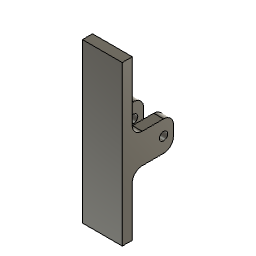
Basis v1 (Autodesk Fusion 360 design; units mm, degrees)
Autodesk Fusion 360 part; units mm, degrees
sketch "Skizze1" plane through (0, 0, 0) normal (1, 0, 0) x (0, 1, 0)
  line L0 (-16.5, 79.8295) -> (-16.5, -80)
  line L1 (-16.5, -80) -> (-6.5, -80)
  line L2 (-6.5, -80) -> (-6.5, -30)
  line L3 (3.5, -20) -> (25, -20)
  arc A0 (3.5, -20) -> (-6.5, -30) centre (3.5, -30) ccw
  line L4 (35, -10) -> (35, 0)
  line L5 (25, 10) -> (3.5, 10)
  line L6 (-6.5, 20) -> (-6.5, 79.9356)
  line L7 (-6.5, 79.9356) -> (-16.5, 79.8295)
  line L8 (-28, -5) -> (49, -5) construction
  line L9 (25, 17) -> (25, -32) construction
  line L10 (-6, -15) -> (-6, -10)
  arc A1 (-6.5, 20) -> (3.5, 10) centre (3.5, 20) ccw
  arc A2 (35, 0) -> (25, 10) centre (25, 0) ccw
  arc A3 (25, -20) -> (35, -10) centre (25, -10) ccw
  circle A4 centre (25, -5) radius 4.15
  point P0 (25, -5)
  dimension "d88" = 80
  dimension "d89" = 10
  dimension "d90" = 10
  dimension "d91" = 5
  dimension "d92" = 25
  dimension "d93" = 35
  dimension "d94" = 15
  dimension "d95" = 15
  dimension "d97" = 31.5
  dimension "d98" = 31
  dimension "d101" = 31.5
  dimension "d102" = 10
  dimension "d103" = 10
  dimension "d104" = 10
  dimension "d105" = 80
  dimension "d106" = 8.3
  constraint vertical L0
  constraint perpendicular L0 L1
  constraint perpendicular L1 L2
  constraint perpendicular L0 L3
  constraint tangent L2 A0
  constraint tangent L3 A0
  constraint perpendicular L3 L4
  constraint perpendicular L4 L5
  constraint perpendicular L5 L6
  constraint horizontal L8
  constraint perpendicular L5 L9
  constraint tangent L5 A1
  constraint tangent L6 A1
  constraint tangent L4 A2
  constraint tangent L5 A2
  constraint tangent L3 A3
  constraint tangent L4 A3
  constraint coincident P0 A4.centre
  measures "d88" distance of L1 origin
  measures "d89" distance of L0 L2
  measures "d90" radius of A0
  measures "d91" distance of origin L8
  measures "d92" distance of origin L9
  measures "d93" distance of origin L4
  measures "d94" distance of L3 L8
  measures "d95" distance of L5 L8
  measures "d97" distance of L2 L9
  measures "d98" distance of L10 P0
  measures "d101" distance of L6 P0
  measures "d102" radius of A1
  measures "d103" radius of A2
  measures "d104" radius of A3
  measures "d105" distance of origin L7
  measures "d106" diameter of A4
extrude "Extrusion1" add sketch "Skizze1" along normal mid plane 40
sketch "Skizze2" plane through (0, 0, -80) normal (0, 0, -1) x (1, 0, 0)
  line L0 (-20, 6.5) -> (20, 6.5)
  line L1 (20, 6.5) -> (20, 16.5)
  line L2 (20, 16.5) -> (-20, 16.5)
  line L3 (-20, 16.5) -> (-20, 6.5)
  line L4 (10.1, -40) -> (-10.1, -40)
  line L5 (-10.1, -40) -> (-10.1, 6.5)
  line L6 (-10.1, 6.5) -> (10.1, 6.5)
  line L7 (10.1, 6.5) -> (10.1, -40)
  dimension "d109" = 10.1
  dimension "d110" = 10.1
  dimension "d111" = 6.5
  dimension "d112" = 40
  constraint horizontal L4
  constraint vertical L5
  constraint horizontal L6
  constraint vertical L7
  measures "d109" distance of origin L5
  measures "d110" distance of origin L7
  measures "d111" distance of origin L6
  measures "d112" distance of origin L4
extrude "Extrusion2" cut sketch "Skizze2" along normal mid plane 200 contours L0 L4 L5 L6 L7
